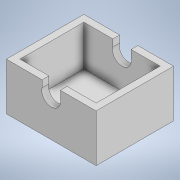
# Autodesk Inventor part: motor_holder#1
Saved by Autodesk Inventor 2021 (Build 250183000, 183)
## iProperties
Created: 2024-03-26
Part Number: motor_holder#1
Material: Generic
Document SubType Name: Modeling
Designer: 23adrdam
Density: 1 g/cm^3
Appearance: Default
Author: 23adrdam
Autodesk Inventor part; units mm, degrees
ref_plane "YZ Plane" through (0, 0, 0) normal (1, 0, 0) x (0, 1, 0)
ref_plane "XZ Plane" through (0, 0, 0) normal (0, 1, 0) x (-1, 0, 0)
ref_plane "XY Plane" through (0, 0, 0) normal (0, 0, 1) x (1, 0, 0)
sketch "Sketch1" plane through (0, 0, 0) normal (0, 1, 0) x (-1, 0, 0)
  line L0 (-11.25, -9.45) -> (11.25, -9.45)
  line L1 (11.25, -9.45) -> (11.25, 9.45)
  line L2 (11.25, 9.45) -> (-11.25, 9.45)
  line L3 (-11.25, 9.45) -> (-11.25, -9.45)
  line L4 (-13.25, -11.45) -> (13.25, -11.45)
  line L5 (13.25, -11.45) -> (13.25, 11.45)
  line L6 (13.25, 11.45) -> (-13.25, 11.45)
  line L7 (-13.25, 11.45) -> (-13.25, -11.45)
  point P0 (0, 0)
  dimension "d0" = 22.5
  dimension "d1" = 18.9
  dimension "d2" = 26.5
  dimension "d3" = 22.9
  dimension "d4" = 9.45
  dimension "d5" = 11.45
  dimension "d6" = 11.25
  dimension "d7" = 13.25
  constraints: 16 end point, 4 parallel, 2 horizontal, 2 perpendicular
  measures "d0" distance of L1.end L2.end
  measures "d1" distance of L0.end L1.end
  measures "d2" distance of L5.end L6.end
  measures "d3" distance of L4.end L5.end
  measures "d4" distance from line of point (0, 0) L0
  measures "d5" distance from line of L4 point (0, 0)
  measures "d6" distance from line of point (0, 0) L3
  measures "d7" distance from line of point (0, 0) L7
extrude "Extrusion1" add sketch "Sketch1" along normal blind 12
sketch "Sketch2" plane through (0, 0, 0) normal (0, -1, 0) x (1, 0, 0)
  line L0 (13.25, -11.45) -> (-13.25, -11.45) projected
  line L1 (13.25, 11.45) -> (-13.25, 11.45)
  line L2 (-13.25, 11.45) -> (-13.25, -11.45)
  line L3 (-13.25, -11.45) -> (13.25, -11.45)
  line L4 (13.25, -11.45) -> (13.25, 11.45)
  line L5 (13.25, 11.45) -> (-13.25, -11.45) construction
  line L6 (-13.25, 11.45) -> (13.25, -11.45) construction
  line L7 (2.5, 2.5) -> (-2.5, 2.5)
  line L8 (-2.5, 2.5) -> (-2.5, -2.5)
  line L9 (-2.5, -2.5) -> (2.5, -2.5)
  line L10 (2.5, -2.5) -> (2.5, 2.5)
  line L11 (2.5, 2.5) -> (-2.5, -2.5) construction
  line L12 (-2.5, 2.5) -> (2.5, -2.5) construction
  point P0 (0, 0)
  dimension "d10" = 5
  dimension "d11" = 5
  constraints: 24 end point, 4 midpoint, 4 parallel, 2 horizontal, 2 perpendicular
  measures "d10" distance of L8.end L9.end
  measures "d11" distance of L7.end L8.end
extrude "Extrusion2" add sketch "Sketch2" along normal blind 2
sketch "Sketch3" plane through (13.25, 12, -11.45) normal (0, 0, -1) x (-1, 0, 0)
  line L0 (10.75, -14) -> (15.75, -14) projected
  line L1 (13.25, -14) -> (13.25, -2.8) construction
  circle A0 centre (13.25, -2.8) radius 2.8
  line L2 (24.5, 0) -> (2, 0) projected
  line L3 (15.95, 0) -> (10.55, 0)
  line L4 (10.55, 0) -> (10.55, -2.8)
  line L5 (10.55, -2.8) -> (15.95, -2.8)
  line L6 (15.95, -2.8) -> (15.95, 0)
  point P0 (13.25, -12)
  point P1 (10.55, -2.0584)
  point P2 (15.95, -2.0584)
  point P3 (10.55, 0)
  dimension "d14" = 11.2
  dimension "d15" = 5.6
  dimension "d16" = 5.4
  dimension "d17" = 2.7
  dimension "d18" = 2.8
  constraints: 10 end point, 2 parallel, 1 centre point, 1 coincident, 1 horizontal, 1 midpoint, 1 perpendicular, 1 point on line, 1 vertical
  measures "d14" distance of L1.start L1.end
  measures "d15" diameter of A0
  measures "d16" distance of L4.end L5.end
  measures "d17" distance between parallel lines of L4 L1
  measures "d18" distance between parallel lines of L2 L5
extrude "Extrusion3" cut sketch "Sketch3" against normal through all
body "Solid1"
